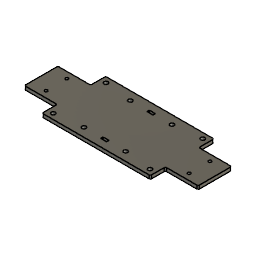
FINAL LFR BOT CHASIS (Autodesk Fusion 360 design; units mm, degrees)
part number: 2026-02-18-15-10-27-309
Autodesk Fusion 360 part; units mm, degrees
sketch "Sketch1" plane through (0, 0, 0) normal (0, 0, 1) x (1, 0, 0)
  line L0 (46.75, 27.5) -> (-46.75, 27.5)
  line L1 (-75, 14.5) -> (-75, -14.5)
  line L2 (-46.75, -27.5) -> (46.75, -27.5)
  line L3 (75, -14.5) -> (75, 14.5)
  line L4 (75, 27.5) -> (-75, -27.5) construction
  line L5 (-75, 27.5) -> (75, -27.5) construction
  line L6 (-46.75, 27.5) -> (-46.75, 14.5)
  line L7 (-46.75, 14.5) -> (-75, 14.5)
  line L8 (46.75, 27.5) -> (46.75, 14.5)
  line L9 (46.75, 14.5) -> (75, 14.5)
  line L10 (-46.75, -27.5) -> (-46.75, -14.5)
  line L11 (-46.75, -14.5) -> (-75, -14.5)
  line L12 (46.75, -27.5) -> (46.75, -14.5)
  line L13 (46.75, -14.5) -> (75, -14.5)
  circle A0 centre (-41.75, 22.75) radius 1.75
  circle A1 centre (41.75, 22.75) radius 1.75
  circle A2 centre (-41.75, -22.75) radius 1.75
  circle A3 centre (41.75, -22.75) radius 1.75
  circle A4 centre (-61.75, 9) radius 1.25
  circle A5 centre (-61.75, -9) radius 1.25
  circle A6 centre (61.75, 9) radius 1.25
  circle A7 centre (61.75, -9) radius 1.25
  circle A8 centre (-18, 20) radius 1.75
  circle A9 centre (18, 20) radius 1.75
  circle A10 centre (-18, -20) radius 1.75
  circle A11 centre (18, -20) radius 1.75
  line L14 (2.5, 21) -> (-2.5, 21)
  line L15 (-2.5, 21) -> (-2.5, 19)
  line L16 (-2.5, 19) -> (2.5, 19)
  line L17 (2.5, 19) -> (2.5, 21)
  line L18 (2.5, 21) -> (-2.5, 19) construction
  line L19 (-2.5, 21) -> (2.5, 19) construction
  line L20 (2.5, -19) -> (-2.5, -19)
  line L21 (-2.5, -19) -> (-2.5, -21)
  line L22 (-2.5, -21) -> (2.5, -21)
  line L23 (2.5, -21) -> (2.5, -19)
  line L24 (2.5, -19) -> (-2.5, -21) construction
  line L25 (-2.5, -19) -> (2.5, -21) construction
  point P0 (0, 20)
  point P1 (0, -20)
  dimension "d1" = 150
  dimension "d2" = 55
  dimension "d3" = 28.25
  dimension "d4" = 13
  dimension "d5" = 28.25
  dimension "d6" = 13
  dimension "d7" = 28.25
  dimension "d8" = 13
  dimension "d9" = 28.25
  dimension "d10" = 13
  dimension "d11" = 3.5
  dimension "d12" = 3.5
  dimension "d13" = 3.5
  dimension "d14" = 3.5
  dimension "d15" = 2.5
  dimension "d16" = 2.5
  dimension "d17" = 2.5
  dimension "d18" = 2.5
  dimension "d19" = 4.75
  dimension "d20" = 5
  dimension "d21" = 5
  dimension "d22" = 4.75
  dimension "d23" = 5
  dimension "d24" = 4.75
  dimension "d25" = 4.75
  dimension "d26" = 5
  dimension "d29" = 13.25
  dimension "d30" = 13.25
  dimension "d33" = 13.25
  dimension "d34" = 13.25
  dimension "d35" = 18
  dimension "d36" = 18
  dimension "d37" = 3.5
  dimension "d38" = 3.5
  dimension "d39" = 3.5
  dimension "d40" = 3.5
  dimension "d41" = 7.5
  dimension "d42" = 7.5
  dimension "d45" = 7.5
  dimension "d46" = 7.5
  dimension "d49" = 5
  dimension "d50" = 2
  dimension "d51" = 5
  dimension "d52" = 2
  constraint horizontal L0
  constraint perpendicular L0 L1
  constraint parallel L0 L2
  constraint parallel L1 L3
  constraint coincident L4 origin
  constraint coincident L5 origin
  constraint vertical L6
  constraint horizontal L7
  constraint vertical L8
  constraint horizontal L9
  constraint vertical L10
  constraint horizontal L11
  constraint vertical L12
  constraint horizontal L13
  constraint horizontal L14
  constraint perpendicular L14 L15
  constraint parallel L14 L16
  constraint parallel L15 L17
  constraint coincident L18 P0
  constraint coincident L19 P0
  constraint horizontal L20
  constraint perpendicular L20 L21
  constraint parallel L20 L22
  constraint parallel L21 L23
  constraint coincident L24 P1
  constraint coincident L25 P1
  measures "d1" distance of L4.end L5.end
  measures "d2" distance of L5.start L4.end
  measures "d3" distance of L5.start L0.end
  measures "d4" distance of L5.start L1.start
  measures "d5" distance of L4.start L0.start
  measures "d6" distance of L4.start L3.end
  measures "d7" distance of L4.end L2.start
  measures "d8" distance of L4.end L1.end
  measures "d9" distance of L5.end L2.end
  measures "d10" distance of L5.end L3.start
  measures "d11" diameter of A0
  measures "d12" diameter of A1
  measures "d13" diameter of A2
  measures "d14" diameter of A3
  measures "d15" diameter of A4
  measures "d16" diameter of A5
  measures "d17" diameter of A6
  measures "d18" diameter of A7
  measures "d19" distance of L2 A2.centre
  measures "d20" distance of L10 A2.centre
  measures "d21" distance of L6 A0.centre
  measures "d22" distance of L0 A0.centre
  measures "d23" distance of L8 A1.centre
  measures "d24" distance of L0 A1.centre
  measures "d25" distance of L2 A3.centre
  measures "d26" distance of L12 A3.centre
  measures "d29" distance of L1 A5.centre
  measures "d30" distance of L1 A4.centre
  measures "d33" distance of L3 A7.centre
  measures "d34" distance of L3 A6.centre
  measures "d35" distance of A4.centre A5.centre
  measures "d36" distance of A6.centre A7.centre
  measures "d37" diameter of A8
  measures "d38" diameter of A9
  measures "d39" diameter of A10
  measures "d40" diameter of A11
  measures "d41" distance of L2 A10.centre
  measures "d42" distance of L2 A11.centre
  measures "d45" distance of L0 A8.centre
  measures "d46" distance of L0 A9.centre
  measures "d49" distance of L15.end L16.end
  measures "d50" distance of L14.end L15.end
  measures "d51" distance of L21.end L22.end
  measures "d52" distance of L20.end L21.end
extrude "Extrude1" add sketch "Sketch1" along normal blind 3
fillet "Fillet1" radius 1 4 edges at (46.75, -27.5, 1.5) (46.75, -14.5, 1.5) (75, -14.5, 1.5) (75, 14.5, 1.5)
fillet "Fillet2" radius 1 8 edges at (46.75, 14.5, 1.5) (46.75, 27.5, 1.5) (-46.75, 27.5, 1.5) (-75, 14.5, 1.5) (-46.75, 14.5, 1.5) (-75, -14.5, 1.5) (-46.75, -27.5, 1.5) (-46.75, -14.5, 1.5)
